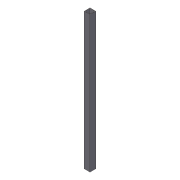
# Autodesk Inventor part: Frame_FrontConveyorGuide
Saved by Autodesk Inventor 2012 (Build 160160000, 160)
## iProperties
Created: 2012-01-21
Part Number: Frame_FrontConveyorGuide
Material: Aluminum-6061
Document SubType Name: Modeling
Designer: JesseK
Mass: 218.575 g
Surface Area: 1019.15 cm^2
Volume: 80.6551 cm^3
Density: 2.71 g/cm^3
Author: JesseK
Autodesk Inventor part; units mm, degrees
ref_plane "YZ Plane" through (0, 0, 0) normal (1, 0, 0) x (0, 1, 0)
ref_plane "XZ Plane" through (0, 0, 0) normal (0, 1, 0) x (-1, 0, 0)
ref_plane "XY Plane" through (0, 0, 0) normal (0, 0, 1) x (1, 0, 0)
sketch "Sketch1" plane through (0, 0, 0) normal (0, 0, 1) x (1, 0, 0)
  line L0 (-243.8061, 206.1329) -> (-243.8061, -327.2671)
  line L1 (-243.8061, -327.2671) -> (-218.4061, -327.2671)
  line L2 (-218.4061, -327.2671) -> (-218.4061, 206.1329)
  line L3 (-218.4061, 206.1329) -> (-243.8061, 206.1329)
  point P0 (0, 0)
  dimension "d1" = 533.4
  dimension "d9" = 25.4
  constraints: 8 end point, 2 horizontal, 2 vertical
  measures "d1" distance of L0.start L0.end
  measures "d9" distance between parallel lines of L2 L0
extrude "Extrusion1" add sketch "Sketch1" along normal blind 25.4
shell "Shell2" thickness 1.5875 removed faces 2 at (-226.8728, -327.2671, 8.4667) at (-235.3394, 206.1329, 8.4667)
body "Solid1"
